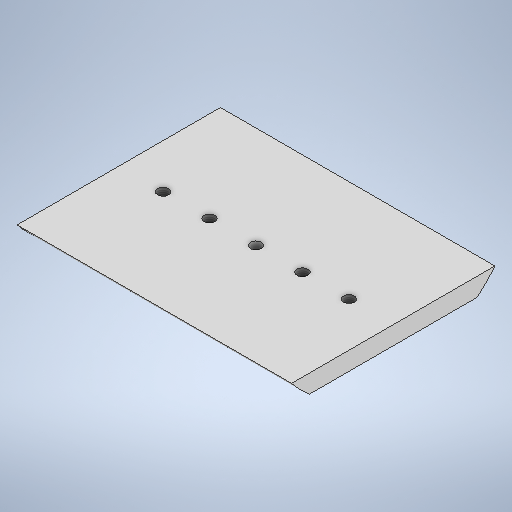
# Autodesk Inventor part: Base
Saved by Autodesk Inventor 2025.3 (Build 293356000, 356)
## iProperties
Created: 2025-05-16
Part Number: Base
Material: Generic
Document SubType Name: Modeling
Designer: Verðandi
Density: 1 g/cm^3
Appearance: Default
Author: Verðandi
Autodesk Inventor part; units mm, degrees
ref_plane "YZ Plane" through (0, 0, 0) normal (1, 0, 0) x (0, 1, 0)
ref_plane "XZ Plane" through (0, 0, 0) normal (0, 1, 0) x (-1, 0, 0)
ref_plane "XY Plane" through (0, 0, 0) normal (0, 0, 1) x (1, 0, 0)
sketch "Sketch1" plane through (0, 0, 0) normal (1, 0, 0) x (0, 1, 0)
  circle A0 centre (0, 0) radius 71
  dimension "d0" = 142
  constraints: 1 centre point, 1 coincident
  measures "d0" diameter of A0
extrude "Extrusion1" add sketch "Sketch1" along normal blind 150
sketch "Sketch2" plane through (150, 0, 0) normal (1, 0, 0) x (0, 0, -1)
  line L0 (0, 0) -> (0, -44.2)
  circle A0 centre (0, 0) radius 71 projected
  line L1 (-55.564, -44.2) -> (55.564, -44.2)
  dimension "d3" = 44.2
  constraints: 4 end point, 2 point on circle, 1 horizontal, 1 vertical
  measures "d3" distance of L0.start L0.end
extrude "Extrusion2" cut sketch "Sketch2" against normal blind 150 contours A0 L1 picked at (-0.2063, 32.437)
sketch "Sketch3" plane through (150, 0, 0) normal (1, 0, 0) x (0, 0, -1)
  line L0 (0, 0) -> (0, -54.2)
  arc A0 (-55.564, -44.2) -> (55.564, -44.2) centre (0, 0) ccw projected
  line L1 (-45.8624, -54.2) -> (45.8624, -54.2)
  dimension "d6" = 54.2
  constraints: 4 end point, 2 point on circle, 1 horizontal, 1 vertical
  measures "d6" distance of L0.start L0.end
extrude "Extrusion3" cut sketch "Sketch3" against normal blind 150
sketch "Sketch6" plane through (150, -44.2, 55.564) normal (0, 1, 0) x (1, 0, 0)
  line L0 (-150, 55.564) -> (-75, 55.564)
  circle A0 centre (-75, 55.564) radius 3
  line L1 (-75, 55.564) -> (-49.6, 55.564)
  line L2 (-49.6, 55.564) -> (-24.2, 55.564)
  line L3 (-75, 55.564) -> (-100.4, 55.564)
  line L4 (-100.4, 55.564) -> (-125.8, 55.564)
  circle A1 centre (-100.4, 55.564) radius 3
  circle A2 centre (-125.8, 55.564) radius 3
  circle A3 centre (-24.2, 55.564) radius 3
  circle A4 centre (-49.6, 55.564) radius 3
  dimension "d51" = 75
  dimension "d52" = 6
  dimension "d53" = 25.4
  dimension "d54" = 25.4
  dimension "d55" = 25.4
  dimension "d56" = 25.4
  dimension "d57" = 6
  dimension "d58" = 6
  dimension "d59" = 6
  dimension "d60" = 6
  constraints: 10 end point, 5 centre point, 5 coincident, 3 point on line, 2 horizontal
  measures "d51" distance of L0.start L0.end
  measures "d52" diameter of A0
  measures "d53" distance of L1.start L1.end
  measures "d54" distance of L1.end L2.end
  measures "d55" distance of L1.start L3.end
  measures "d56" distance of L3.end L4.end
  measures "d57" diameter of A1
  measures "d58" diameter of A2
  measures "d59" diameter of A3
  measures "d60" diameter of A4
extrude "Extrusion4" cut sketch "Sketch6" against normal blind 10
thread "Thread1" size "M6x1" class "6H" standard "ANSI Metric M Profile" full length
thread "Thread2" size "M6x1" class "6H" standard "ANSI Metric M Profile" full length
thread "Thread3" size "M6x1" class "6H" standard "ANSI Metric M Profile" full length
thread "Thread4" size "M6x1" class "6H" standard "ANSI Metric M Profile" full length
body "Solid1"
